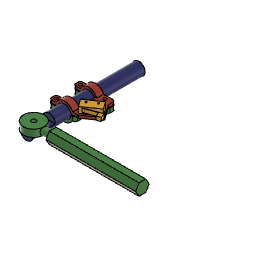
Limitswitch_steering_holder (Autodesk Fusion 360 design; units mm, degrees)
Autodesk Fusion 360 part; units mm, degrees
sketch "Sketch1" plane through (0, 0, 0) normal (0, 0, 1) x (1, 0, 0) in component "limitswitch"
  line L0 (10, 5) -> (-10, 5)
  line L1 (-10, 5) -> (-10, -5)
  line L2 (-10, -5) -> (10, -5)
  line L3 (10, -5) -> (10, 5)
  line L4 (10, 5) -> (-10, -5) construction
  line L5 (-10, 5) -> (10, -5) construction
  circle A0 centre (5, -2) radius 1
  circle A1 centre (-5, -2) radius 1
  dimension "d1" = 20
  dimension "d2" = 10
  dimension "d3" = 2
  dimension "d4" = 2
  dimension "d5" = 3
  dimension "d6" = 5
  dimension "d7" = 5
  constraint horizontal L0
  constraint perpendicular L0 L1
  constraint parallel L0 L2
  constraint parallel L1 L3
  constraint coincident L4 origin
  constraint coincident L5 origin
  constraint horizontal A0.centre A1.centre
  measures "d1" distance of L1.end L2.end
  measures "d2" distance of L0.end L1.end
  measures "d3" diameter of A0
  measures "d4" diameter of A1
  measures "d5" distance of L2 A0.centre
  measures "d6" distance of L3 A0.centre
  measures "d7" distance of L1 A1.centre
extrude "Extrude1" add sketch "Sketch1" along normal blind 6.5 makes body 1 in component "limitswitch"
sketch "Sketch2" plane through (0, -5, 0) normal (0, -1, 0) x (1, 0, 0) in component "limitswitch"
  line L0 (-10, 0) -> (10, 0)
  line L1 (10, 0) -> (10, 6.5)
  line L2 (10, 6.5) -> (-10, 6.5)
  line L3 (-10, 6.5) -> (-10, 0)
  line L4 (-8, 1.75) -> (-9, 1.75)
  line L5 (-9, 1.75) -> (-9, 4.75)
  line L6 (-9, 4.75) -> (-8, 4.75)
  line L7 (-8, 4.75) -> (-8, 1.75)
  line L8 (-8, 1.75) -> (-9, 4.75) construction
  line L9 (-9, 1.75) -> (-8, 4.75) construction
  line L10 (-10, 3.7764) -> (-10, 3.5051)
  line L11 (10, 3.25) -> (-10, 3.25) construction
  line L12 (0.5, 1.75) -> (-0.5, 1.75)
  line L13 (0.5, 1.75) -> (-0.5, 4.75) construction
  line L14 (-0.5, 4.75) -> (0.5, 4.75)
  line L15 (0.5, 4.75) -> (0.5, 1.75)
  line L16 (-0.5, 1.75) -> (0.5, 4.75) construction
  line L17 (-0.5, 1.75) -> (-0.5, 4.75)
  line L18 (9, 1.75) -> (8, 1.75)
  line L19 (9, 1.75) -> (8, 4.75) construction
  line L20 (8, 4.75) -> (9, 4.75)
  line L21 (9, 4.75) -> (9, 1.75)
  line L22 (8, 1.75) -> (9, 4.75) construction
  line L23 (8, 1.75) -> (8, 4.75)
  point P0 (-8.5, 3.25)
  point P1 (0, 3.25)
  point P2 (8.5, 3.25)
  dimension "d10" = 1
  dimension "d11" = 3
  dimension "d12" = 1
  dimension "d13" = 3
  dimension "d14" = 1
  dimension "d15" = 3
  dimension "d16" = 1.5
  dimension "d17" = 1.5
  constraint horizontal L4
  constraint perpendicular L4 L5
  constraint parallel L4 L6
  constraint parallel L5 L7
  constraint coincident L8 P0
  constraint coincident L9 P0
  constraint coincident L3 L10.start
  constraint midpoint L1 L11.start
  constraint midpoint L3 L11.end
  constraint horizontal L12
  constraint perpendicular L12 L17
  constraint parallel L12 L14
  constraint parallel L15 L17
  constraint coincident P1 L13
  constraint coincident P1 L16
  constraint horizontal L18
  constraint perpendicular L18 L23
  constraint parallel L18 L20
  constraint parallel L21 L23
  constraint coincident P2 L19
  constraint coincident P2 L22
  constraint midpoint L11 P1
  constraint coincident L11 P2
  measures "d10" distance of L5.end L6.end
  measures "d11" distance of L4.end L5.end
  measures "d12" distance of L13.end L14.end
  measures "d13" distance of L12.end L13.end
  measures "d14" distance of L19.end L20.end
  measures "d15" distance of L18.end L19.end
  measures "d16" distance of L1 P2
  measures "d17" distance of L3 P0
extrude "Extrude2" add sketch "Sketch2" along normal blind 4 contours L4 L5 L6 L7 | L12 L14 L15 L17 | L18 L20 L21 L23 bodies 1 in component "limitswitch"
ref_plane "WorkPlane1" through (0, 0, 3.25) normal (0, 0, 1) x (1, 0, 0) in component "limitswitch"
sketch "Sketch3" plane through (0, 0, 3.25) normal (0, 0, 1) x (1, 0, 0) in component "limitswitch"
  circle A0 centre (5, -2) radius 1
  circle A1 centre (-5, -2) radius 1
  line L0 (10, -5) -> (10, 5)
  line L1 (10, 5) -> (-10, 5)
  line L2 (-10, 5) -> (-10, -5)
  line L3 (-10, -5) -> (10, -5)
  line L4 (-7, 5) -> (11.3526, 9.9176)
  line L5 (11.3526, 9.9176) -> (10.0585, 14.7472)
  line L6 (10.0585, 14.7472) -> (5.7118, 13.5825)
  line L7 (5.7118, 13.5825) -> (7.0059, 8.7529)
  line L8 (11.3526, 9.9176) -> (11.482, 9.4346)
  line L9 (11.482, 9.4346) -> (-5.0681, 5)
  dimension "d20" = 19
  dimension "d21" = 3
  dimension "d22" = 4.5
  dimension "d23" = 0.5
  dimension "d24" = 15
  dimension "d25" = 5
  constraint coincident L1 L4.start
  constraint perpendicular L4 L5
  constraint coincident L4 L7.end
  constraint perpendicular L4 L7
  constraint perpendicular L4 L8
  constraint coincident L1 L9.end
  constraint parallel L4 L9
  constraint perpendicular L5 L6
  measures "d20" distance of L4.start L4.end
  measures "d21" distance of L2 L4.start
  measures "d22" distance of L5 L7
  measures "d23" distance of L4 L9
  measures "d24" angle of L1 L4
  measures "d25" distance of L4 L6
extrude "Extrude3" add sketch "Sketch3" along normal blind 2 and the other way blind 2 contours L1 L4 L8 L9 | L4 L5 L6 L7 bodies 1 in component "limitswitch"
sketch "Sketch1 (2)" plane through (0, 0, 0) normal (0, 0, 1) x (1, 0, 0) in component "tube_clamp"
  circle A0 centre (0, 0) radius 15
  circle A1 centre (0, 0) radius 15.5
  line L0 (38.2121, 0) -> (-34.1582, 0) construction
  circle A2 centre (0, 0) radius 20.5
  line L1 (26, 0) -> (26, -5)
  line L2 (26, -5) -> (19.8809, -5)
  line L3 (26, -1) -> (20.4756, -1)
  line L4 (-20.4756, -1) -> (-35.4756, -1)
  line L5 (-35.4756, -1) -> (-35.4756, -5)
  line L6 (-35.4756, -5) -> (-19.8809, -5)
  line L7 (-20.4756, -1) -> (-15.4677, -1)
  line L8 (20.4756, -1) -> (15.4677, -1)
  line L9 (20.4756, 1) -> (26, 1)
  line L10 (26, 1) -> (26, 5)
  line L11 (26, 5) -> (19.8809, 5)
  line L12 (-20.4756, 1) -> (-26, 1)
  line L13 (-26, 1) -> (-26, 5)
  line L14 (-26, 5) -> (-19.8809, 5)
  line L15 (20.4756, 1) -> (15.4677, 1)
  line L16 (-20.4756, 1) -> (-15.4677, 1)
  dimension "d30" = 30
  dimension "d32" = 0.5
  dimension "d33" = 5
  dimension "d34" = 26
  dimension "d36" = 1
  dimension "d37" = 4
  dimension "d38" = 1
  dimension "d39" = 4
  dimension "d40" = 15
  dimension "d56" = 26
  dimension "d57" = 1
  dimension "d58" = 4
  dimension "d59" = 26
  dimension "d60" = 1
  dimension "d61" = 4
  constraint coincident A0.centre A1.centre
  constraint horizontal L0
  constraint coincident A0.centre L0
  constraint concentric A1 A2
  constraint coincident L0 L1.start
  constraint perpendicular L0 L1
  constraint coincident A2 L2.end
  constraint perpendicular L1 L2
  constraint coincident L1 L3.start
  constraint coincident A2 L3.end
  constraint perpendicular L1 L3
  constraint coincident A2 L4.start
  constraint parallel L0 L4
  constraint perpendicular L0 L5
  constraint coincident A2 L6.end
  constraint perpendicular L5 L6
  constraint coincident A1 L7.end
  constraint parallel L4 L7
  constraint coincident A1 L8.end
  constraint parallel L3 L8
  constraint coincident A2 L9.start
  constraint parallel L0 L9
  constraint perpendicular L9 L10
  constraint coincident A2 L11.end
  constraint perpendicular L10 L11
  constraint coincident A2 L12.start
  constraint horizontal L12
  constraint perpendicular L12 L13
  constraint coincident A2 L14.end
  constraint perpendicular L13 L14
  constraint coincident A1 L15.end
  constraint parallel L0 L15
  constraint coincident A1 L16.end
  constraint parallel L12 L16
  measures "d30" diameter of A0
  measures "d32" distance of A0 A1
  measures "d33" distance of A1 A2
  measures "d34" distance of A0.centre L1
  measures "d36" distance of L0 L3
  measures "d37" distance of L2 L3
  measures "d38" distance of L0 L4
  measures "d39" distance of L4 L6
  measures "d40" distance of L4.start L5
  measures "d56" distance of A0.centre L10
  measures "d57" distance of L0 L9
  measures "d58" distance of L9 L11
  measures "d59" distance of A0.centre L13
  measures "d60" distance of L0 L12
  measures "d61" distance of L12 L14
extrude "Extrude1'" add sketch "Sketch1 (2)" along normal blind 5 and the other way blind 5 separate body contours A1 A2 L7 L8 | A2 L1 L2 L3 | A2 L4 L5 L6 makes body 2 in component "tube_clamp"
extrude "Extrude4" add sketch "Sketch1 (2)" along normal blind 5 and the other way blind 5 separate body contours A1 A2 L15 L16 | A2 L9 L10 L11 | A2 L12 L13 L14 makes body 3 in component "tube_clamp"
sketch "Sketch2 (2)" plane through (0, -5, 0) normal (0, -1, 0) x (1, 0, 0) in component "tube_clamp"
  line L0 (26, -5) -> (26, 5)
  line L1 (26, 5) -> (19.8809, 5)
  line L2 (19.8809, 5) -> (19.8809, -5)
  line L3 (19.8809, -5) -> (26, -5)
  line L4 (-19.8809, -5) -> (-19.8809, 5)
  line L5 (-19.8809, 5) -> (-35.4756, 5)
  line L6 (-35.4756, 5) -> (-35.4756, -5)
  line L7 (-35.4756, -5) -> (-19.8809, -5)
  circle A0 centre (-22.8809, 0) radius 1.75
  circle A1 centre (22.8809, 0) radius 1.75
  dimension "d45" = 3.5
  dimension "d46" = 3.5
  dimension "d47" = 3
  dimension "d48" = 3
  constraint horizontal A0.centre A1.centre
  constraint horizontal origin A1.centre
  measures "d45" diameter of A0
  measures "d46" diameter of A1
  measures "d47" distance of L2 A1.centre
  measures "d48" distance of L4 A0.centre
extrude "Extrude2'" cut sketch "Sketch2 (2)" against normal blind 19 contours A0 | A1 bodies 2 3 in component "tube_clamp"
sketch "Sketch4" plane through (0, 5, 0) normal (0, 1, 0) x (-1, 0, 0) in component "tube_clamp"
  circle A0 centre (22.8809, 0) radius 1.75
  line L0 (26, -5) -> (26, 5)
  line L1 (26, 5) -> (19.8809, 5)
  line L2 (19.8809, 5) -> (19.8809, -5)
  line L3 (19.8809, -5) -> (26, -5)
  circle A1 centre (-22.8809, 0) radius 1.75
  line L4 (-19.8809, -5) -> (-19.8809, 5)
  line L5 (-19.8809, 5) -> (-26, 5)
  line L6 (-26, 5) -> (-26, -5)
  line L7 (-26, -5) -> (-19.8809, -5)
  line L8 (25.7309, 1.6454) -> (22.8809, 3.2909)
  line L9 (22.8809, 3.2909) -> (20.0309, 1.6454)
  line L10 (20.0309, 1.6454) -> (20.0309, -1.6454)
  line L11 (20.0309, -1.6454) -> (22.8809, -3.2909)
  line L12 (22.8809, -3.2909) -> (25.7309, -1.6454)
  line L13 (25.7309, -1.6454) -> (25.7309, 1.6454)
  line L14 (-22.8809, 3.2909) -> (-25.7309, 1.6454)
  line L15 (-25.7309, 1.6454) -> (-25.7309, -1.6454)
  line L16 (-25.7309, -1.6454) -> (-22.8809, -3.2909)
  line L17 (-22.8809, -3.2909) -> (-20.0309, -1.6454)
  line L18 (-20.0309, -1.6454) -> (-20.0309, 1.6454)
  line L19 (-20.0309, 1.6454) -> (-22.8809, 3.2909)
  point P0 (22.8809, 0)
  point P1 (-22.8809, 0)
  dimension "d66" = 2.85
  dimension "d67" = 2.85
  constraint coincident P0 A0.centre
  constraint coincident P1 A1.centre
  constraint parallel L4 L18
  constraint parallel L2 L13
  measures "d66" distance of P0 L13
  measures "d67" distance of P1 L19
extrude "Extrude5" cut sketch "Sketch4" against normal blind 2.5 contours L8 L9 L10 L11 L12 L13 | L14 L15 L16 L17 L18 L19 bodies 3 in component "tube_clamp"
sketch "Sketch3 (2)" plane through (0, -5, 0) normal (0, -1, 0) x (1, 0, 0) in component "tube_clamp"
  circle A0 centre (-22.8809, 0) radius 1.75
  line L0 (-19.8809, -5) -> (-19.8809, 5)
  line L1 (-19.8809, 5) -> (-35.4756, 5)
  line L2 (-35.4756, 5) -> (-35.4756, -5)
  line L3 (-35.4756, -5) -> (-19.8809, -5)
  line L4 (-35.4756, -5) -> (-35.4756, -13)
  line L5 (-35.4756, -13) -> (-20.4756, -13)
  line L6 (-35.4756, 0) -> (-33.4756, 0) construction
  line L7 (-20.4756, -13) -> (-20.4756, 5)
  dimension "d84" = 18
  dimension "d85" = 15
  constraint coincident L2.end L3.start
  constraint perpendicular L3 L4
  constraint perpendicular L4 L5
  constraint midpoint L2 L6.start
  constraint coincident L1 L7.end
  constraint perpendicular L1 L7
  measures "d84" distance of L1 L5
  measures "d85" distance of L2 L7
extrude "Extrude3'" add sketch "Sketch3 (2)" against normal up to surface (4 mm away) contours L3 L4 L5 L7 | L1 L2 L3 L7 bodies 2 in component "tube_clamp"
sketch "Sketch5" plane through (0, -5, 0) normal (0, -1, 0) x (1, 0, 0) in component "tube_clamp"
  line L0 (-19.8809, -5) -> (-19.8809, 5)
  line L1 (-19.8809, 5) -> (-35.4756, 5)
  line L2 (-35.4756, 5) -> (-35.4756, -13)
  line L3 (-35.4756, -13) -> (-20.4756, -13)
  line L4 (-20.4756, -5) -> (-19.8809, -5)
  circle A0 centre (-31.4756, -9) radius 1
  circle A1 centre (-31.4756, 1) radius 1
  line L5 (-33.4756, -10.25) -> (-28.4756, -10.25)
  arc A2 (-28.4756, -10.25) -> (-28.4756, -7.75) centre (-28.4756, -9) ccw
  line L6 (-28.4756, -7.75) -> (-33.4756, -7.75)
  arc A3 (-33.4756, -7.75) -> (-33.4756, -10.25) centre (-33.4756, -9) ccw
  line L7 (-33.4756, -9) -> (-28.4756, -9) construction
  line L8 (-28.4756, 2.25) -> (-33.4756, 2.25)
  arc A4 (-33.4756, 2.25) -> (-33.4756, -0.25) centre (-33.4756, 1) ccw
  line L9 (-33.4756, -0.25) -> (-28.4756, -0.25)
  arc A5 (-28.4756, -0.25) -> (-28.4756, 2.25) centre (-28.4756, 1) ccw
  line L10 (-28.4756, 1) -> (-33.4756, 1) construction
  line L11 (-20.4756, -13) -> (-20.4756, -5)
  circle A6 centre (-22.8809, 0) radius 1.75
  dimension "d74" = 2.5
  dimension "d75" = 2.5
  dimension "d76" = 2
  dimension "d79" = 2
  dimension "d86" = 7
  constraint tangent L5 A2
  constraint tangent A2 L6
  constraint parallel L5 L6
  constraint tangent L6 A3
  constraint tangent L5 A3
  constraint horizontal L7
  constraint tangent L8 A4
  constraint tangent A4 L9
  constraint parallel L8 L9
  constraint tangent L9 A5
  constraint tangent L8 A5
  constraint horizontal L10
  constraint coincident A1.centre L10
  constraint coincident A0.centre L7
  constraint vertical A2.centre A5.centre
  measures "d74" diameter of A2
  measures "d75" diameter of A4
  measures "d76" distance of L2 A3.centre
  measures "d79" distance of L2 A4.centre
  measures "d86" distance of L2 A2.centre
extrude "Extrude6" cut sketch "Sketch5" against normal blind 5 contours A0 | A1 | L5 A2 L6 A3 | L8 A4 L9 A5 bodies 2 in component "tube_clamp"
fillet "Fillet1" radius 3 16 edges at (-35.4756, -3, -13) (-15.4677, -1, 0) (15.4677, -1, 0) (26, -3, 5) (26, -3, -5) (-35.4756, -3, 5) (-20.4756, -3, -5) (-20.4756, -3, -13) (-26, 3, -5) (-26, 3, 5) (-19.8809, 5, 0) (26, 3, -5) (26, 3, 5) (19.8809, 5, 0) (15.4677, 1, 0) (-15.4677, 1, 0) on bodies 2 3 in component "tube_clamp"
sketch "Sketch1 (3)" plane through (0, 0, 0) normal (0, 0, 1) x (1, 0, 0) in component "connection_rod"
  circle A0 centre (0, 0) radius 2.5
  circle A1 centre (0, 0) radius 11.5
  dimension "d87" = 5
  dimension "d88" = 23
  constraint coincident A0.centre A1.centre
  measures "d87" diameter of A0
  measures "d88" diameter of A1
extrude "Extrude1''" add sketch "Sketch1 (3)" along normal blind 4 and the other way blind 4 separate body makes body 4 in component "connection_rod"
sketch "Sketch2 (3)" plane through (0, 0, 0) normal (1, 0, 0) x (0, 1, 0) in component "connection_rod"
  circle A0 centre (0, 0) radius 4
  dimension "d93" = 8
  constraint coincident A0.centre origin
  measures "d93" diameter of A0
extrude "Extrude2''" add sketch "Sketch2 (3)" along normal blind 16 from surface at 5 bodies 4 in component "connection_rod"
sketch "Sketch3 (3)" plane through (21, 0, 0) normal (1, 0, 0) x (0, 1, 0) in component "connection_rod"
  circle A0 centre (0, 0) radius 4
  line L0 (-3.7528, 6.5) -> (-7.5056, 0)
  line L1 (-7.5056, 0) -> (-3.7528, -6.5)
  line L2 (-3.7528, -6.5) -> (3.7528, -6.5)
  line L3 (3.7528, -6.5) -> (7.5056, 0)
  line L4 (7.5056, 0) -> (3.7528, 6.5)
  line L5 (3.7528, 6.5) -> (-3.7528, 6.5)
  line L6 (11.5, 4) -> (-11.5, 4)
  dimension "d97" = 6.5
  constraint coincident A0.centre origin
  constraint parallel L5 L6
  measures "d97" distance of A0.centre L5
extrude "Extrude3''" add sketch "Sketch3 (3)" along normal blind 100 contours A0 | L0 L1 L2 L3 L4 L6 | L0 L4 L5 L6 bodies 4 in component "connection_rod"
sketch "Sketch1 (4)" plane through (0, 0, 0) normal (0, 1, 0) x (1, 0, 0) in component "swiwel_connection"
  circle A0 centre (0, 0) radius 7
  dimension "d100" = 14
  constraint coincident A0.centre origin
  measures "d100" diameter of A0
extrude "Extrude1'''" add sketch "Sketch1 (4)" along normal blind 100 separate body makes body 5 in component "swiwel_connection"
sketch "Sketch2 (4)" plane through (0, 0, 0) normal (0, 0, 1) x (1, 0, 0) in component "swiwel_connection"
  line L0 (7, 100) -> (-7, 100)
  line L1 (7, 0) -> (-7, 0)
  line L2 (7, 0) -> (-7, 0)
  line L3 (-7, 0) -> (-7, -25)
  line L4 (-7, -25) -> (7, -25)
  line L5 (7, -25) -> (7, 0)
  circle A0 centre (0, -17) radius 2.5
  dimension "d103" = 25
  dimension "d104" = 5
  dimension "d105" = 17
  constraint horizontal L2
  constraint vertical L3
  constraint horizontal L4
  constraint vertical L5
  constraint coincident L1.start L2.start
  constraint vertical origin A0.centre
  measures "d103" distance of L1.start L4.end
  measures "d104" diameter of A0
  measures "d105" distance of L2 A0.centre
extrude "Extrude2'''" add sketch "Sketch2 (4)" against normal blind 7 bodies 5 in component "swiwel_connection"
fillet "Fillet1'" radius 7 2 edges at (-7, -12.5, -7) (7, -12.5, -7) on bodies 5 in component "swiwel_connection"
fillet "Fillet1'" radius 5 2 edges at (7, -25, -3.5) (-7, -25, -3.5) on bodies 5 in component "swiwel_connection"
sketch "Sketch1 (5)" plane through (0, 0, 0) normal (0, 0, 1) x (1, 0, 0) in component "limitswitch_holder_top"
  line L0 (18.5842, 37.9015) -> (34.6848, 43.7617)
  line L1 (30.6272, 41.7527) -> (17.0017, 36.7934)
  line L2 (32.3373, 37.0543) -> (30.6272, 41.7527)
  line L3 (36.566, 38.5934) -> (32.3373, 37.0543)
  line L4 (34.6848, 43.7617) -> (36.566, 38.5934)
  line L5 (23.5532, 53.5886) -> (21.2589, 56.8652)
  line L6 (22.0781, 57.4388) -> (21.2589, 56.8652)
  line L7 (24.3724, 54.1622) -> (22.0781, 57.4388)
  line L8 (16.5904, 48.7132) -> (14.2961, 51.9898)
  line L9 (15.1153, 52.5634) -> (14.2961, 51.9898)
  line L10 (17.4096, 49.2868) -> (15.1153, 52.5634)
  line L11 (10.4468, 44.4114) -> (8.1525, 47.688)
  line L12 (9.6276, 43.8378) -> (7.3333, 47.1144)
  line L13 (8.1525, 47.688) -> (7.3333, 47.1144)
  circle A0 centre (14.625, 43.6747) radius 1
  circle A1 centre (22.8165, 49.4104) radius 1
  line L14 (8.8085, 43.2642) -> (9.6276, 43.8378)
  line L15 (10.4468, 44.4114) -> (16.5904, 48.7132)
  line L16 (17.4096, 49.2868) -> (23.5532, 53.5886)
  line L17 (24.3724, 54.1622) -> (25.1915, 54.7358)
  line L18 (14.5442, 35.0727) -> (8.8085, 43.2642)
  line L19 (30.9273, 46.5442) -> (18.5842, 37.9015)
  line L20 (17.0017, 36.7934) -> (14.5442, 35.0727)
  line L21 (25.1915, 54.7358) -> (30.9273, 46.5442)
  line L22 (18.5842, 37.9015) -> (17.0017, 36.7934)
  line L23 (7, -8) -> (-7, -8)
  spline S0 degree 3 poles (0, -2.5) (0.3169, -2.5) (0.653, -2.4361) (1.2682, -2.1801) (1.5474, -1.9881) (1.9882, -1.5473) (2.1801, -1.2681) (2.4361, -0.6531) (2.5, -0.3171) (2.5, 0) (2.5, 0.3171) (2.4361, 0.6531) (2.1801, 1.2681) (1.9882, 1.5473) (1.5474, 1.9881) (1.2682, 2.1801) (0.653, 2.4361) (0.3169, 2.5) (0, 2.5) knots 1.141051 1.141051 1.141051 1.141051 1.236109 1.236109 1.331167 1.331167 1.426284 1.426284 1.521401 1.521401 1.521401 1.616518 1.616518 1.711635 1.711635 1.806693 1.806693 1.901751 1.901751 1.901751 1.901751
  spline S1 degree 3 poles (0, 2.5) (-0.3169, 2.5) (-0.653, 2.4361) (-1.2682, 2.1801) (-1.5474, 1.9881) (-1.9882, 1.5473) (-2.1801, 1.2681) (-2.4361, 0.6531) (-2.5, 0.3171) (-2.5, 0) (-2.5, -0.3171) (-2.4361, -0.6531) (-2.1801, -1.2681) (-1.9882, -1.5473) (-1.5474, -1.9881) (-1.2682, -2.1801) (-0.653, -2.4361) (-0.3169, -2.5) (0, -2.5) knots 1.141051 1.141051 1.141051 1.141051 1.236109 1.236109 1.331167 1.331167 1.426284 1.426284 1.521401 1.521401 1.521401 1.616518 1.616518 1.711635 1.711635 1.806693 1.806693 1.901751 1.901751 1.901751 1.901751
  line L24 (7, -8) -> (7, 17)
  line L25 (-7, 17) -> (-7, -8)
  line L26 (7, 117) -> (-7, 117)
  line L27 (7, 17) -> (7, 117)
  line L28 (-7, 17) -> (-7, 117)
  line L29 (14.8595, 34.0727) -> (7, 34.0727)
  line L30 (14.8595, 34.0727) -> (32.32, 46.2987)
  line L31 (32.32, 46.2987) -> (22, 61.0372)
  line L32 (22, 61.0372) -> (22, 68.5372)
  line L33 (22, 68.5372) -> (7, 68.5372)
  line L34 (26.7083, 46.0316) -> (22.1197, 52.5849)
  arc A2 (22.1197, 52.5849) -> (20.0718, 51.1509) centre (21.0958, 51.8679) ccw
  line L35 (20.0718, 51.1509) -> (24.6604, 44.5977)
  arc A3 (24.6604, 44.5977) -> (26.7083, 46.0316) centre (25.6844, 45.3147) ccw
  line L36 (25.6844, 45.3147) -> (21.0958, 51.8679) construction
  line L37 (18.5168, 40.2959) -> (13.9282, 46.8491)
  arc A4 (13.9282, 46.8491) -> (11.8803, 45.4151) centre (12.9042, 46.1321) ccw
  line L38 (11.8803, 45.4151) -> (16.4689, 38.8619)
  arc A5 (16.4689, 38.8619) -> (18.5168, 40.2959) centre (17.4929, 39.5789) ccw
  line L39 (18.2098, 38.555) -> (12.1873, 47.1561) construction
  circle A6 centre (14.5, 64.7872) radius 1.75
  line L40 (7.25, 34.0727) -> (7.25, 68.5372)
  circle A7 centre (12.25, 38.0727) radius 1.75
  dimension "d130" = 1
  dimension "d131" = 1
  dimension "d132" = 1
  dimension "d133" = 15
  dimension "d134" = 7.5
  dimension "d135" = 2.5
  dimension "d136" = 2.5
  dimension "d137" = 8
  dimension "d138" = 3
  dimension "d139" = 3
  dimension "d140" = 8
  dimension "d141" = 3.5
  dimension "d142" = 7.5
  dimension "d143" = 3.75
  dimension "d146" = 0.25
  dimension "d158" = 3.5
  dimension "d159" = 5
  dimension "d160" = 4
  constraint coincident L0.start L19.end
  constraint coincident L1.end L20.start
  constraint coincident L27 L29.end
  constraint perpendicular L27 L29
  constraint perpendicular L30 L31
  constraint perpendicular L29 L32
  constraint coincident L27 L33.end
  constraint perpendicular L27 L33
  constraint parallel L19 L30
  constraint tangent L34 A2
  constraint tangent A2 L35
  constraint parallel L34 L35
  constraint tangent L35 A3
  constraint tangent L34 A3
  constraint perpendicular L19 L36
  constraint coincident A1.centre L36
  constraint tangent L37 A4
  constraint tangent A4 L38
  constraint parallel L37 L38
  constraint tangent L38 A5
  constraint tangent L37 A5
  constraint midpoint A5 L39.start
  constraint midpoint A4 L39.end
  constraint coincident A0.centre L39
  constraint parallel L35 L37
  constraint coincident L29 L40.start
  constraint coincident L33 L40.end
  constraint perpendicular L33 L40
  measures "d130" distance of L19 L30
  measures "d131" distance of L21 L31
  measures "d132" distance of L18.start L29
  measures "d133" distance of L27 L32.end
  measures "d134" distance of L31.end L33
  measures "d135" diameter of A2
  measures "d136" diameter of A4
  measures "d137" distance of A5.centre A4.centre
  measures "d138" distance of L30 A5.centre
  measures "d139" distance of L30 A3.centre
  measures "d140" distance of A3.centre A2.centre
  measures "d141" diameter of A6
  measures "d142" distance of L32 A6.centre
  measures "d143" distance of L33 A6.centre
  measures "d146" distance of L27 L40
  measures "d158" diameter of A7
  measures "d159" distance of L40 A7.centre
  measures "d160" distance of L29 A7.centre
extrude "Extrude2''''" add sketch "Sketch1 (5)" against normal blind 3 separate body contours L0 L1 L5 L6 L7 L8 L9 L10 L11 L12 L13 L14 L15 L16 L17 L18 L19 L20 L21 L29 L30 L31 L32 L33 A2 A4 L40 A7 | L5 L6 L7 L8 L9 L10 L11 L12 L13 L14 L15 L16 L17 L18 L19 L20 L21 L22 L34 L35 A3 L37 L38 A5 A7 | L0 L1 L22 L30 | L18 A7 | L18 A7 makes body 6 in component "limitswitch_holder_top"
sketch "Sketch2 (5)" plane through (0, 68.5372, 0) normal (0, 1, 0) x (-1, 0, 0) in component "limitswitch_holder_top"
  line L0 (-7.25, 0) -> (-22, 0)
  line L1 (-22, 0) -> (-22, -3)
  line L2 (-22, -3) -> (-7.25, -3)
  line L3 (-7.25, -3) -> (-7.25, 0)
  arc A0 (-7, -4) -> (7, -4) centre (0, -4) ccw
  arc A1 (7, -4) -> (-7, -4) centre (0, -4) ccw
  arc A2 (7.25, -4) -> (-7.25, -4) centre (0, -4) ccw
  arc A3 (-7.25, -4) -> (7.25, -4) centre (0, -4) ccw
  circle A4 centre (0, -4) radius 10
  line L4 (-7.25, 0) -> (-6.0467, 0)
  line L5 (-7.25, -3) -> (-7.1807, -3)
  line L6 (7.1807, -3) -> (9.9499, -3)
  line L7 (6.0467, 0) -> (9.1652, 0)
  line L8 (9.1652, 0) -> (16.6652, 0)
  line L9 (9.9499, -3) -> (16.6652, -3)
  line L10 (16.6652, -3) -> (16.6652, 0)
  line L11 (-32.32, 0) -> (-32.32, -3)
  line L12 (-7.25, 0) -> (-7.25, -3)
  line L13 (-14.8595, 0) -> (-7.25, 0)
  line L14 (-14.8595, -3) -> (-7.25, -3)
  line L15 (-14.8595, 0) -> (-32.32, 0)
  line L16 (-32.32, -3) -> (-14.8595, -3)
  dimension "d147" = 0.25
  dimension "d148" = 20
  dimension "d149" = 7.5
  constraint concentric A0 A4
  constraint coincident L0.start L3.end
  constraint coincident A2 L4.end
  constraint perpendicular L3 L4
  constraint coincident L2.end L3.start
  constraint coincident A3 L5.end
  constraint perpendicular L3 L5
  constraint coincident A3 L6.start
  constraint coincident A4 L6.end
  constraint parallel L5 L6
  constraint coincident L2.end L6
  constraint coincident A2 L7.start
  constraint coincident A4 L7.end
  constraint horizontal L7
  constraint coincident L4.end L7
  constraint parallel L7 L8
  constraint parallel L6 L9
  constraint perpendicular L9 L10
  measures "d148" diameter of A4
  measures "d149" distance of L7.end L8.end
extrude "Extrude3'''" add sketch "Sketch2 (5)" against normal up to surface (7.5 mm away) contours L0 A2 A4 L4 L7 L13 | L3 A2 L4 L5 L12 | A4 L8 L9 L10 | A2 A4 L6 L7 bodies 6 in component "limitswitch_holder_top"
extrude "Extrude4'" add sketch "Sketch2 (5)" along normal blind 7.5 from surface at -34.4645 contours L0 A2 A4 L4 L7 L13 | L3 A2 L4 L5 L12 | A4 L8 L9 L10 | A2 A4 L6 L7 bodies 6 in component "limitswitch_holder_top"
sketch "Sketch3 (4)" plane through (0, 0, 0) normal (0, 0, 1) x (-1, 0, 0) in component "limitswitch_holder_top"
  line L0 (16.6652, -61.0372) -> (9.1652, -61.0372)
  line L1 (9.1652, -61.0372) -> (9.1652, -68.5372)
  line L2 (9.1652, -68.5372) -> (16.6652, -68.5372)
  line L3 (16.6652, -68.5372) -> (16.6652, -61.0372)
  line L4 (16.6652, -34.0727) -> (9.1652, -34.0727)
  line L5 (9.1652, -34.0727) -> (9.1652, -41.5727)
  line L6 (9.1652, -41.5727) -> (16.6652, -41.5727)
  line L7 (16.6652, -41.5727) -> (16.6652, -34.0727)
  circle A0 centre (12.9152, -37.8227) radius 1.75
  circle A1 centre (12.9152, -64.7872) radius 1.75
  dimension "d161" = 3.5
  dimension "d162" = 3.5
  measures "d161" diameter of A0
  measures "d162" diameter of A1
extrude "Extrude6'" cut sketch "Sketch3 (4)" against normal blind 5 contours A0 | A1 bodies 6 in component "limitswitch_holder_top"
fillet "Fillet1''" radius 2 11 edges at (-16.6652, 68.5372, -1.5) (-16.6652, 61.0372, -1.5) (-16.6652, 41.5727, -1.5) (-16.6652, 34.0727, -1.5) (22, 68.5372, -1.5) (32.32, 46.2987, -1.5) (14.8595, 34.0727, -1.5) (-7.1807, 37.8227, -3) (-7.1807, 64.7872, -3) (7.1807, 64.7872, -3) (7.1807, 37.8227, -3) on bodies 6 in component "limitswitch_holder_top"
ref_plane "WorkPlane1" through (20.535, 51.3049, -4) normal (0, 0, -1) x (-1, 0, 0) in component "limittswitch_bottom_holder"
sketch "Sketch1 (6)" plane through (20.535, 51.3049, -4) normal (0, 0, -1) x (1, 0, 0) in component "limittswitch_bottom_holder"
  line L0 (-11.785, 17.2322) -> (-11.785, -17.2322)
  line L1 (-11.785, -17.2322) -> (-0.535, -17.2322)
  arc A0 (-0.535, -17.2322) -> (1.465, -15.2322) centre (-0.535, -15.2322) ccw
  line L2 (1.465, -15.2322) -> (1.465, -9.7322)
  line L3 (1.465, -9.7322) -> (10.6379, 3.368)
  arc A1 (10.6379, 3.368) -> (10.1467, 6.1534) centre (8.9995, 4.5151) ccw
  line L4 (10.1467, 6.1534) -> (-5.1589, 16.8705)
  arc A2 (-5.1589, 16.8705) -> (-6.3061, 17.2322) centre (-6.3061, 15.2322) ccw
  line L5 (-6.3061, 17.2322) -> (-11.785, 17.2322)
  arc A3 (6.1733, 5.2733) -> (4.1254, 6.7072) centre (5.1494, 5.9903) ccw
  line L6 (6.1733, 5.2733) -> (1.5847, -1.2799)
  arc A4 (-0.4632, 0.154) -> (1.5847, -1.2799) centre (0.5608, -0.5629) ccw
  line L7 (-0.4632, 0.154) -> (4.1254, 6.7072)
  circle A5 centre (-6.035, -13.4822) radius 1.75
  arc A6 (-2.0182, 11.0091) -> (-4.0661, 12.443) centre (-3.0422, 11.726) ccw
  line L8 (-2.0182, 11.0091) -> (-6.6068, 4.4559)
  arc A7 (-8.6547, 5.8898) -> (-6.6068, 4.4559) centre (-7.6308, 5.1728) ccw
  line L9 (-8.6547, 5.8898) -> (-4.0661, 12.443)
  line L10 (-29.285, -17.2322) -> (-29.285, -9.7322)
  line L11 (-29.285, -9.7322) -> (-35.2002, -9.7322)
  arc A8 (-35.2002, -9.7322) -> (-37.2002, -11.7322) centre (-35.2002, -11.7322) ccw
  line L12 (-37.2002, -11.7322) -> (-37.2002, -15.2322)
  arc A9 (-37.2002, -15.2322) -> (-35.2002, -17.2322) centre (-35.2002, -15.2322) ccw
  line L13 (-35.2002, -17.2322) -> (-29.285, -17.2322)
  circle A10 centre (-33.4502, -13.4822) radius 1.75
  line L14 (-29.285, 9.7322) -> (-29.285, 17.2322)
  line L15 (-29.285, 17.2322) -> (-35.2002, 17.2322)
  arc A11 (-35.2002, 17.2322) -> (-37.2002, 15.2322) centre (-35.2002, 15.2322) ccw
  line L16 (-37.2002, 15.2322) -> (-37.2002, 11.7322)
  arc A12 (-37.2002, 11.7322) -> (-35.2002, 9.7322) centre (-35.2002, 11.7322) ccw
  line L17 (-35.2002, 9.7322) -> (-29.285, 9.7322)
  circle A13 centre (-33.4502, 13.4822) radius 1.75
  line L18 (-27.535, 59.3049) -> (-13.535, 59.3049)
  line L19 (-27.535, 59.3049) -> (-27.535, 34.3049)
  line L20 (-27.535, 34.3049) -> (-13.535, 34.3049)
  line L21 (-13.535, 34.3049) -> (-13.535, 59.3049)
  line L22 (-27.535, -65.6951) -> (-13.535, -65.6951)
  spline S0 degree 3 poles (-20.535, 53.8049) (-20.2181, 53.8049) (-19.882, 53.7411) (-19.2668, 53.485) (-18.9876, 53.293) (-18.5468, 52.8522) (-18.3549, 52.573) (-18.0989, 51.958) (-18.035, 51.622) (-18.035, 51.3049) (-18.035, 50.9879) (-18.0989, 50.6518) (-18.3549, 50.0369) (-18.5468, 49.7576) (-18.9876, 49.3168) (-19.2668, 49.1249) (-19.882, 48.8688) (-20.2181, 48.8049) (-20.535, 48.8049) knots 1.141051 1.141051 1.141051 1.141051 1.236109 1.236109 1.331167 1.331167 1.426284 1.426284 1.521401 1.521401 1.521401 1.616518 1.616518 1.711635 1.711635 1.806693 1.806693 1.901751 1.901751 1.901751 1.901751
  spline S1 degree 3 poles (-20.535, 48.8049) (-20.8519, 48.8049) (-21.188, 48.8688) (-21.8032, 49.1249) (-22.0824, 49.3168) (-22.5232, 49.7576) (-22.7151, 50.0369) (-22.9711, 50.6518) (-23.035, 50.9879) (-23.035, 51.3049) (-23.035, 51.622) (-22.9711, 51.958) (-22.7151, 52.573) (-22.5232, 52.8522) (-22.0824, 53.293) (-21.8032, 53.485) (-21.188, 53.7411) (-20.8519, 53.8049) (-20.535, 53.8049) knots 1.141051 1.141051 1.141051 1.141051 1.236109 1.236109 1.331167 1.331167 1.426284 1.426284 1.521401 1.521401 1.521401 1.616518 1.616518 1.711635 1.711635 1.806693 1.806693 1.901751 1.901751 1.901751 1.901751
  line L23 (-27.535, 59.3049) -> (-13.535, 59.3049)
  circle A14 centre (-20.535, 51.3049) radius 2.5
  line L24 (-13.535, 59.3049) -> (-13.535, 34.3049)
  line L25 (-27.535, 34.3049) -> (-27.535, 59.3049)
  line L26 (-27.535, -65.6951) -> (-13.535, -65.6951)
  line L27 (-27.535, 34.3049) -> (-27.535, -65.6951)
  line L28 (-13.535, 34.3049) -> (-13.535, -65.6951)
  line L29 (-11.785, -17.2322) -> (-13.535, -17.2322)
  line L30 (-29.285, -17.2322) -> (-27.535, -17.2322)
  line L31 (-29.285, -9.7322) -> (-27.535, -9.7322)
  line L32 (-29.285, 17.2322) -> (-27.535, 17.2322)
  line L33 (-29.285, 9.7322) -> (-27.535, 9.7322)
  line L34 (-11.785, 17.2322) -> (-13.535, 17.2322)
  line L35 (-13.285, 34.3049) -> (-13.285, -65.9451)
  line L36 (-27.785, -65.9451) -> (-13.285, -65.9451)
  line L37 (-27.785, 34.3049) -> (-27.785, -65.9451)
  line L38 (-27.785, 34.3049) -> (-27.785, 59.5549)
  line L39 (-27.785, 59.5549) -> (-13.285, 59.5549)
  line L40 (-13.285, 59.5549) -> (-13.285, 34.3049)
  line L41 (-13.285, -9.7322) -> (-11.785, -9.7322)
  line L42 (-13.285, 9.7322) -> (-11.785, 9.7322)
  line L43 (1.465, -9.7322) -> (-8.785, -3.8144)
  line L44 (-8.785, 17.2322) -> (-8.785, -3.8144)
  dimension "d197" = 0.25
  dimension "d212" = 3
  dimension "d213" = 120
  constraint coincident L0.end L1.start
  constraint coincident L28 L29.end
  constraint perpendicular L28 L29
  constraint coincident L10.start L13.end
  constraint coincident L27 L30.end
  constraint perpendicular L27 L30
  constraint coincident L10.end L11.start
  constraint coincident L27 L31.end
  constraint perpendicular L27 L31
  constraint coincident L14.end L15.start
  constraint coincident L27 L32.end
  constraint perpendicular L27 L32
  constraint coincident L14.start L17.end
  constraint coincident L27 L33.end
  constraint perpendicular L27 L33
  constraint coincident L0.start L5.end
  constraint coincident L28 L34.end
  constraint perpendicular L0 L34
  constraint coincident L35 L41.start
  constraint coincident L0 L41.end
  constraint perpendicular L0 L41
  constraint coincident L35 L42.start
  constraint coincident L0 L42.end
  constraint perpendicular L0 L42
  constraint coincident L33.end L42
  constraint coincident L31.end L41
  constraint coincident L2.end L3.start
  constraint coincident L5 L44.start
  constraint perpendicular L5 L44
  measures "d212" distance of L0 L44
  measures "d213" angle of L43 L44
extrude "Extrude1''''" add sketch "Sketch1 (6)" along normal blind 5 separate body contours L0 L1 A0 L2 L5 A7 L43 L44 | L0 L34 L35 L42 | L0 L29 L35 L41 | A7 L44 | L14 L32 L33 L37 | L10 L30 L31 L37 | L14 L15 A11 L16 A12 L17 | L10 L11 A8 L12 A9 L13 makes body 7 at (16.2964, 59.7716, -4) makes body 8 at (-8.5551, 64.7872, -4) makes body 9 at (-8.5551, 37.8227, -4) in component "limittswitch_bottom_holder"
sketch "Sketch2 (6)" plane through (0, 34.0727, 0) normal (0, -1, 0) x (1, 0, 0) in component "limittswitch_bottom_holder"
  line L0 (11.75, -4) -> (7.25, -4)
  line L1 (7.25, -4) -> (7.25, -9)
  line L2 (7.25, -9) -> (11.75, -9)
  circle A0 centre (0, -4) radius 7
  line L3 (-7.25, -4) -> (-7.25, -9)
  line L4 (-14.6652, -4) -> (-7.25, -4)
  line L5 (-14.6652, -9) -> (-7.25, -9)
  line L6 (-16.6652, -4) -> (-14.6652, -4)
  line L7 (-16.6652, -9) -> (-14.6652, -9)
  line L8 (-16.6652, -4) -> (-16.6652, -9)
  line L9 (7.25, -4) -> (7.25, -9)
  line L10 (20, -4) -> (22, -4)
  line L11 (20, -9) -> (22, -9)
  line L12 (20, -4) -> (7.25, -4)
  line L13 (7.25, -9) -> (20, -9)
  circle A1 centre (0, -4) radius 7.3
  circle A2 centre (0, -4) radius 10
  line L14 (22, -4) -> (22, -9)
  line L15 (11.75, -9) -> (11.75, -4)
  dimension "d200" = 0.3
  dimension "d201" = 20
  constraint concentric A0 A2
  measures "d201" diameter of A2
extrude "Extrude2'''''" add sketch "Sketch2 (6)" against normal up to surface (7.5 mm away) contours L1 L2 L3 L5 L9 L13 A1 A2 bodies 7 9 in component "limittswitch_bottom_holder"
extrude "Extrude3''''" add sketch "Sketch2 (6)" along normal up to surface (7.5 mm away) from surface at -34.4645 contours L1 L2 L3 L5 L9 L13 A1 A2 bodies 7 8 in component "limittswitch_bottom_holder"
sketch "Sketch3 (5)" plane through (0, 0, -9) normal (0, 0, -1) x (1, 0, 0) in component "limittswitch_bottom_holder"
  circle A0 centre (14.5, -64.7872) radius 1.75
  line L0 (8.6603, -61.0372) -> (8.6603, -68.5372)
  line L1 (8.6603, -68.5372) -> (20, -68.5372)
  arc A1 (20, -68.5372) -> (22, -66.5372) centre (20, -66.5372) ccw
  line L2 (22, -66.5372) -> (22, -61.0372)
  line L3 (11.75, -34.0727) -> (8.6603, -34.0727)
  line L4 (8.6603, -34.0727) -> (8.6603, -41.5727)
  line L5 (8.6603, -41.5727) -> (8.75, -41.5727)
  line L6 (8.75, -41.5727) -> (8.75, -61.0372)
  line L7 (8.75, -61.0372) -> (8.6603, -61.0372)
  line L8 (-8.6603, -41.5727) -> (-8.6603, -34.0727)
  line L9 (-8.6603, -34.0727) -> (-14.6652, -34.0727)
  arc A2 (-14.6652, -34.0727) -> (-16.6652, -36.0727) centre (-14.6652, -36.0727) ccw
  line L10 (-16.6652, -36.0727) -> (-16.6652, -39.5727)
  arc A3 (-16.6652, -39.5727) -> (-14.6652, -41.5727) centre (-14.6652, -39.5727) ccw
  line L11 (-14.6652, -41.5727) -> (-8.6603, -41.5727)
  circle A4 centre (-12.9152, -37.8227) radius 1.75
  line L12 (-8.6603, -68.5372) -> (-8.6603, -61.0372)
  line L13 (-8.6603, -61.0372) -> (-14.6652, -61.0372)
  arc A5 (-14.6652, -61.0372) -> (-16.6652, -63.0372) centre (-14.6652, -63.0372) ccw
  line L14 (-16.6652, -63.0372) -> (-16.6652, -66.5372)
  arc A6 (-16.6652, -66.5372) -> (-14.6652, -68.5372) centre (-14.6652, -66.5372) ccw
  line L15 (-14.6652, -68.5372) -> (-8.6603, -68.5372)
  circle A7 centre (-12.9152, -64.7872) radius 1.75
  line L16 (-11.2697, -40.6727) -> (-9.6243, -37.8227)
  line L17 (-9.6243, -37.8227) -> (-11.2697, -34.9727)
  line L18 (-11.2697, -34.9727) -> (-14.5606, -34.9727)
  line L19 (-14.5606, -34.9727) -> (-16.206, -37.8227)
  line L20 (-16.206, -37.8227) -> (-14.5606, -40.6727)
  line L21 (-14.5606, -40.6727) -> (-11.2697, -40.6727)
  line L22 (-11.2697, -67.6372) -> (-9.6243, -64.7872)
  line L23 (-9.6243, -64.7872) -> (-11.2697, -61.9372)
  line L24 (-11.2697, -61.9372) -> (-14.5606, -61.9372)
  line L25 (-14.5606, -61.9372) -> (-16.206, -64.7872)
  line L26 (-16.206, -64.7872) -> (-14.5606, -67.6372)
  line L27 (-14.5606, -67.6372) -> (-11.2697, -67.6372)
  line L28 (16.1454, -67.6372) -> (17.7909, -64.7872)
  line L29 (17.7909, -64.7872) -> (16.1454, -61.9372)
  line L30 (16.1454, -61.9372) -> (12.8546, -61.9372)
  line L31 (12.8546, -61.9372) -> (11.2091, -64.7872)
  line L32 (11.2091, -64.7872) -> (12.8546, -67.6372)
  line L33 (12.8546, -67.6372) -> (16.1454, -67.6372)
  line L34 (22, -61.0372) -> (11.75, -55.1193)
  line L35 (11.75, -55.1193) -> (11.75, -34.0727)
  point P0 (-12.9152, -37.8227)
  point P1 (-12.9152, -64.7872)
  point P2 (14.5, -64.7872)
  dimension "d207" = 2.85
  dimension "d208" = 2.85
  dimension "d209" = 2.85
  constraint coincident P0 A4.centre
  constraint coincident P1 A7.centre
  constraint parallel L15 L27
  constraint parallel L11 L21
  constraint coincident P2 A0.centre
  constraint parallel L1 L33
  measures "d207" distance of P0 L21
  measures "d208" distance of P1 L27
  measures "d209" distance of P2 L33
extrude "Extrude4''" cut sketch "Sketch3 (5)" against normal blind 3 contours L16 L17 L18 L19 L20 L21 | L22 L23 L24 L25 L26 L27 | L28 L29 L30 L31 L32 L33 bodies 7 in component "limittswitch_bottom_holder"
fillet "Fillet1'''" radius 3 3 edges at (22, 61.0372, -6.5) (11.75, 55.1193, -6.5) (11.75, 34.0727, -6.5) on bodies 7 in component "limittswitch_bottom_holder"
ref_plane "WorkPlane1" through (0, 117, -4) normal (0, 1, 0) x (1, 0, 0) in component "clamp_bottom"
sketch "Sketch1 (7)" plane through (0, 117, -4) normal (0, 1, 0) x (1, 0, 0) in component "clamp_bottom"
  line L0 (19, -4) -> (19, 1)
  line L1 (19, 1) -> (7.1807, 1)
  arc A0 (-7.1807, 1) -> (7.1807, 1) centre (0, 0) ccw
  line L2 (-7.1807, 1) -> (-11.2488, 1)
  line L3 (-11.2488, -4) -> (-9.1652, -4)
  arc A1 (-9.1652, -4) -> (9.1652, -4) centre (0, 0) ccw
  line L4 (9.1652, -4) -> (19, -4)
  line L5 (-14.5815, -4) -> (-16.6652, -4)
  line L6 (-16.6652, 1) -> (-14.5815, 1)
  line L7 (-16.6652, 1) -> (-16.6652, -4)
  circle A2 centre (0, 0) radius 7
  circle A3 centre (0, 0) radius 7.25
  line L8 (-16.6652, 2) -> (-16.6652, 7)
  circle A4 centre (0, 0) radius 10
  line L9 (-16.6652, 7) -> (-7.1414, 7)
  line L10 (7.1414, 7) -> (19.2824, 7)
  line L11 (19.2824, 7) -> (19.2824, 2)
  line L12 (19.2824, 2) -> (9.798, 2)
  line L13 (-16.6652, 2) -> (-6.9687, 2)
  line L14 (9.798, 2) -> (6.9687, 2)
  line L15 (16.4531, 2) -> (16.4531, 7)
  line L16 (-11.2488, 1) -> (-11.2488, -4)
  line L17 (-14.5815, -4) -> (-14.5815, 1)
  dimension "d168" = 9.4844
  dimension "d169" = 0.25
  dimension "d170" = 20
  dimension "d171" = 1
  dimension "d172" = 5
  dimension "d173" = 5
  dimension "d174" = 9.4844
  dimension "d177" = 9.4844
  constraint concentric A0 A4
  constraint coincident A4 L9.end
  constraint perpendicular L8 L9
  constraint coincident A4 L10.start
  constraint parallel L9 L10
  constraint coincident A4 L12.end
  constraint parallel L10 L12
  constraint coincident A3 L13.end
  constraint perpendicular L8 L13
  constraint coincident L6.start L8
  constraint perpendicular L10 L11
  constraint coincident L12 L13.end
  constraint coincident L9 L10.end
  constraint coincident A3 L14.end
  constraint parallel L12 L14
  constraint coincident L12 L15.start
  constraint coincident L10 L15.end
  constraint perpendicular L10 L15
  measures "d168" distance of A0.start L6.start
  measures "d170" diameter of A4
  measures "d171" distance of L6 L13
  measures "d172" distance of L5.start L6.end
  measures "d173" distance of L8.start L8.end
  measures "d174" distance of L11.end L12.end
  measures "d177" distance of L14.end L15
component "no work" placed x (1, 0, 0) y (0, 1, 0) z (0, 0, 1) at (0, 0, 0)
component "should_work" placed x (1, 0, 0) y (0, 1, 0) z (0, 0, 1) at (0, 0, 0)
component "limitswitch" placed x (0, 0, -1) y (-1, 0, 0) z (0, 1, 0) at (-33.4756, -12.5, -4) in component "no work"
component "tube_clamp" placed x (1, 0, 0) y (0, 1, 0) z (0, 0, 1) at (0, 0, 0) in component "no work"
component "swiwel_connection" placed x (1, 0, 0) y (0, 1, 0) z (0, 0, 1) at (0, 17, -4) in component "should_work"
component "connection_rod" placed x (1, 0, 0) y (0, 1, 0) z (0, 0, 1) at (0, 0, 0) in component "should_work"
component "limitswitch" placed x (0.819152, 0.573576, 0) y (0.573576, -0.819152, 0) z (0, 0, -1) at (19.8679, 44.9042, 7.5) in component "should_work"
component "limitswitch_holder_top" placed x (1, 0, 0) y (0, 1, 0) z (0, 0, 1) at (0, 0, 0) in component "should_work"
component "limittswitch_bottom_holder" placed x (1, 0, 0) y (0, 1, 0) z (0, 0, 1) at (0, 0, 0) in component "should_work"
equation "d56 = d34"
equation "d57 = d36"
equation "d58 = d37"
equation "d59 = d34"
equation "d60 = d57"
equation "d61 = d37"
equation "d95 = 21 mm - 5 mm"
equation "d97 = ( 13 / 2 ) * 1 mm"
equation "d142 = d133 / 2"
equation "d143 = d134 / 2"
equation "d173 = d172"
equation "d174 = d168"
equation "d177 = d168"
named bodies: "Upper_clamp", "Lower_clamp"
